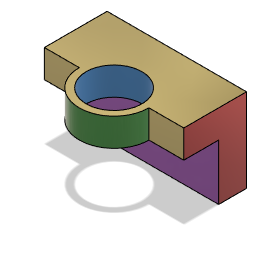
Questão2 (Autodesk Fusion 360 design; units mm, degrees)
Autodesk Fusion 360 part; units mm, degrees
sketch "Sketch1" plane through (0, 0, 0) normal (0, 0, 1) x (1, 0, 0)
  line L0 (-60, 70) -> (40, 70)
  line L1 (40, 70) -> (40, 10)
  line L2 (40, 10) -> (-60, 10)
  line L3 (-60, 10) -> (-60, 70)
  line L4 (-60, 70) -> (40, 70)
  line L5 (40, 70) -> (40, 50)
  line L6 (40, 50) -> (-60, 50)
  line L7 (-60, 50) -> (-60, 70)
  line L8 (-60, 70) -> (-35, 70)
  line L9 (-35, 70) -> (15, 70)
  line L10 (15, 70) -> (15, 50)
  line L11 (15, 50) -> (-35, 50)
  line L12 (-35, 50) -> (-35, 70)
  dimension "d1" = 100
  dimension "d2" = 60
  constraint horizontal L0
  constraint vertical L1
  constraint horizontal L2
  constraint vertical L3
  constraint horizontal L4
  constraint vertical L5
  constraint horizontal L6
  constraint vertical L7
  constraint coincident L1 L5.end
  constraint coincident L4 L8.end
  constraint horizontal L9
  constraint vertical L10
  constraint horizontal L11
  constraint vertical L12
  constraint coincident L6 L10.end
  measures "d1" distance of L0.start L0.end
  measures "d2" distance of L0.start L2.end
extrude "Extrude1" add sketch "Sketch1" along normal blind 20 contours L1 L2 L3 L6 L11
extrude "Extrude2" add sketch "Sketch1" along normal blind 45 contours L0 L3 L4 L6 L7 L8 L12
extrude "Extrude3" add sketch "Sketch1" along normal blind 45 contours L0 L1 L4 L5 L6 L10
extrude "Extrude4" add sketch "Sketch1" along normal blind 45 contours L0 L4 L6 L9 L10 L11 L12
sketch "Sketch2" plane through (0, 50, 0) normal (0, -1, 0) x (1, 0, 0)
  line L0 (-60, 20) -> (40, 20)
  line L1 (40, 20) -> (40, 45)
  line L2 (40, 45) -> (-60, 45)
  line L3 (-60, 45) -> (-60, 20)
sketch "Sketch3" plane through (0, 50, 0) normal (0, -1, 0) x (1, 0, 0)
  line L0 (-35, 45) -> (-30, 45)
  circle A0 centre (-10, 45) radius 20
  line L1 (10, 45) -> (15, 45)
  arc A1 (15, 45) -> (-35, 45) centre (-10, 45) ccw
  dimension "d12" = 40
  dimension "d13" = 50
  constraint horizontal L0
  constraint parallel L0 L1
  constraint coincident A0 L0.end
  constraint coincident A0 L1.start
  measures "d12" diameter of A0
  measures "d13" diameter of A1
hole "Hole1" at (-10, 50, 45) direction (0, 1, 0) diameter 40 depth 600 tip angle 118
extrude "Extrude5" add sketch "Sketch3" against normal blind 20 contours L0 A0 L1 A1
